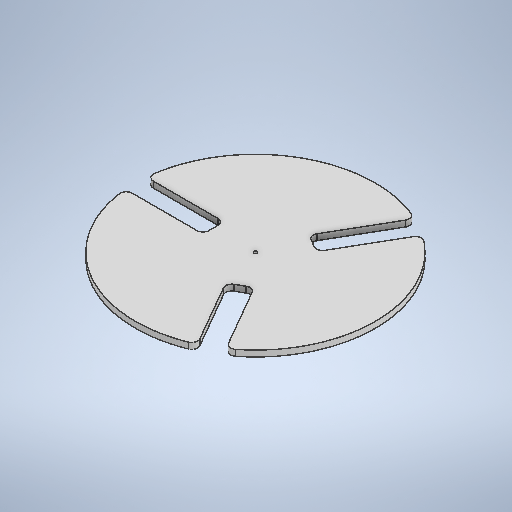
# Autodesk Inventor part: RT_FRM_V2_MC_004_TopDynamicsPlate
Saved by Autodesk Inventor 2025.3 (Build 293356000, 356)
## iProperties
Created: 2026-04-28
Part Number: RT_FRM_V2_MC_004_TopDynamicsPlate
Material: Generic
Document SubType Name: Modeling
Designer: louis
Density: 1 g/cm^3
Appearance: Default
Mass: 556.266 g
Surface Area: 1307.88 cm^2
Volume: 556.266 cm^3
Author: louis
Autodesk Inventor part; units mm, degrees
ref_plane "YZ Plane" through (0, 0, 0) normal (1, 0, 0) x (0, 1, 0)
ref_plane "XZ Plane" through (0, 0, 0) normal (0, 1, 0) x (-1, 0, 0)
ref_plane "XY Plane" through (0, 0, 0) normal (0, 0, 1) x (1, 0, 0)
sketch "Sketch1" plane through (0, 0, 0) normal (0, 1, 0) x (-1, 0, 0)
  line L0 (30, -2.5) -> (140, -2.5)
  line L1 (185, 0) -> (25, 0)
  line L2 (0, 0) -> (25, 0)
  circle A0 centre (0, 0) radius 200
  line L3 (50, 0) -> (103.8137, 0) construction
  line L4 (105, 16.5) -> (105, 0) construction
  line L5 (105, 66.5) -> (105, 16.5) construction
  line L6 (199.2329, -17.5) -> (70, -17.5)
  line L7 (70, -17.5) -> (70, 17.5)
  line L8 (70, 17.5) -> (199.2329, 17.5)
  line L9 (199.2329, 17.5) -> (199.2329, -17.5)
  line L10 (0, 0) -> (0, 200)
  line L11 (-64.9519, 112.5) -> (0, 0)
  circle A1 centre (0, 0) radius 310 construction
  line L12 (-310, -390) -> (-310, -310) construction
  line L13 (-310, -310) -> (-390, -310) construction
  line L14 (-390, -310) -> (-390, -390) construction
  line L15 (-390, -390) -> (-310, -390) construction
  line L16 (-310, -390) -> (-390, -310) construction
  line L17 (-310, -310) -> (-390, -390) construction
  line L18 (-310, 310) -> (-310, 390) construction
  line L19 (-310, 390) -> (-390, 390) construction
  line L20 (-390, 390) -> (-390, 310) construction
  line L21 (-390, 310) -> (-310, 310) construction
  line L22 (-310, 310) -> (-390, 390) construction
  line L23 (-310, 390) -> (-390, 310) construction
  line L24 (390, 310) -> (390, 390) construction
  line L25 (390, 390) -> (310, 390) construction
  line L26 (310, 390) -> (310, 310) construction
  line L27 (310, 310) -> (390, 310) construction
  line L28 (390, 310) -> (310, 390) construction
  line L29 (390, 390) -> (310, 310) construction
  line L30 (390, -390) -> (390, -310) construction
  line L31 (390, -310) -> (310, -310) construction
  line L32 (310, -310) -> (310, -390) construction
  line L33 (310, -390) -> (390, -390) construction
  line L34 (390, -390) -> (310, -310) construction
  line L35 (390, -310) -> (310, -390) construction
  line L36 (310, -310) -> (310, 310) construction
  line L37 (310, 310) -> (-310, 310) construction
  line L38 (-310, 310) -> (-310, -310) construction
  line L39 (-310, -310) -> (310, -310) construction
  line L40 (-64.9519, 112.5) -> (-100, 173.2051)
  line L41 (160, 17.5) -> (199.2329, 17.5)
  line L42 (-114.7719, 163.7908) -> (-84.461, 181.2908)
  line L43 (-84.461, -181.2908) -> (-114.7719, -163.7908)
  point P0 (188.2651, -67.5)
  point P1 (70, 0)
  point P2 (-84.461, 181.2908)
  point P3 (-99.6165, 172.5408)
  point P4 (199.2329, 0)
  point P5 (-114.7719, 163.7908)
  point P6 (-84.461, -181.2908)
  point P7 (-114.7719, -163.7908)
  dimension "d0" = 110
  dimension "d2" = 2.5
  dimension "d4" = 105
  dimension "d9" = 400
  dimension "d26" = 35
  dimension "d27" = 35
  dimension "d40" = 50
  dimension "d46" = 120
  dimension "d74" = 80
  dimension "d75" = 80
  dimension "d78" = 80
  dimension "d79" = 80
  dimension "d80" = 80
  dimension "d81" = 80
  dimension "d82" = 80
  dimension "d83" = 80
  dimension "d86" = 620
  dimension "d97" = 360
  constraints: 88 end point, 10 parallel, 10 perpendicular, 6 vertical, 5 point on circle, 3 coincident, 3 horizontal, 3 point on line, 3 tangent, 2 centre point, 2 collinear, 1 midpoint, 10 other
  measures "d0" distance of L0.end L0.start
  measures "d2" distance between parallel lines of L0 L1
  measures "d4" distance of L2.start L4.end
  measures "d9" diameter of A0
  measures "d26" distance between parallel lines of L8 L6
  measures "d27" distance between parallel lines of L4 L7
  measures "d40" distance from line of L6 point (188.265, -67.5)
  measures "d46" angle of L11 L2
  measures "d74" distance of L13.end L14.end
  measures "d75" distance of L14.end L12.start
  measures "d78" distance of L19.end L20.end
  measures "d79" distance of L20.end L18.start
  measures "d80" distance of L25.end L26.end
  measures "d81" distance of L26.end L24.start
  measures "d82" distance of L31.end L32.end
  measures "d83" distance of L32.end L30.start
  measures "d86" distance of L26.end L18.start
extrude "Extrusion1" add sketch "Sketch1" against normal blind 10 contours L1 L2 L10 A0 L8 L7 | L11 L40 L42 A0 L10 | A0 L43
pattern_circular "Circular Pattern2" count 3 over 360 about axis through (0, 0, 0) along (0, -1, 0) of "Extrusion1"
extrude "Extrusion2" cut sketch "Sketch1" against normal blind 10 contours L7 L8 L9 L6 | L9 A0
pattern_circular "Circular Pattern1" count 3 over 360 about axis through (0, -10, 0) along (0, 1, 0) of "Extrusion2"
fillet "Fillet1" radius 10 6 edges at (19.8446, -5, 69.3718) (50.1554, -5, -51.8718) (-70, -5, -17.5) (-70, -5, 17.5) (50.1554, -5, 51.8718) (19.8446, -5, -69.3718)
sketch "Sketch2" plane through (0, -10, 0) normal (0, 1, 0) x (1, 0, 0)
  line L0 (20, 310) -> (-20, 310) construction
  line L1 (-20, 310) -> (-20, -310) construction
  line L2 (-20, -310) -> (20, -310) construction
  line L3 (20, -310) -> (20, 310) construction
  line L4 (20, 310) -> (-20, -310) construction
  line L5 (-20, 310) -> (20, -310) construction
  line L6 (60, 20) -> (20, 20) construction
  line L7 (20, 20) -> (20, -20) construction
  line L8 (20, -20) -> (60, -20) construction
  line L9 (60, -20) -> (60, 20) construction
  line L10 (60, 20) -> (20, -20) construction
  line L11 (20, 20) -> (60, -20) construction
  line L12 (-60, 123.6771) -> (-20, 123.6771) construction
  line L13 (-20, 123.6771) -> (-20, 83.6771) construction
  line L14 (-20, 83.6771) -> (-60, 83.6771) construction
  line L15 (-60, 83.6771) -> (-60, 123.6771) construction
  line L16 (-60, 123.6771) -> (-20, 83.6771) construction
  line L17 (-20, 123.6771) -> (-60, 83.6771) construction
  line L18 (-60, -66.8914) -> (-20, -66.8914) construction
  line L19 (-20, -66.8914) -> (-20, -106.8914) construction
  line L20 (-20, -106.8914) -> (-60, -106.8914) construction
  line L21 (-60, -106.8914) -> (-60, -66.8914) construction
  line L22 (-60, -66.8914) -> (-20, -106.8914) construction
  line L23 (-20, -66.8914) -> (-60, -106.8914) construction
  point P0 (0, 0)
  point P1 (40, 0)
  point P2 (-40, 103.6771)
  point P3 (-40, -86.8914)
  dimension "d87" = 40
  dimension "d88" = 620
  dimension "d89" = 40
  dimension "d90" = 40
  dimension "d91" = 40
  dimension "d92" = 40
  dimension "d93" = 40
  dimension "d94" = 40
  constraints: 48 end point, 8 midpoint, 8 parallel, 4 horizontal, 4 perpendicular, 3 collinear
  measures "d87" distance of L2.end L1.end
  measures "d88" distance of L1.end L0.end
  measures "d89" distance of L8.end L7.end
  measures "d90" distance of L7.end L6.end
  measures "d91" distance of L13.end L14.end
  measures "d92" distance of L19.end L20.end
  measures "d93" distance of L18.end L19.end
  measures "d94" distance of L14.end L12.start
hole "Hole2" [suppressed]
sketch "Sketch3" plane through (0, -10, 0) normal (0, -1, 0) x (1, 0, 0)
  point P0 (0, 0)
  point P1 (0, 0)
  constraints: 1 coincident
hole "Hole3" at (0, -10, 0) direction (0, 1, 0) diameter 5.5 end through all start extended yes counterbore diameter 10 counterbore depth 5 clearance for "Socket Head Cap Screw" size "M5" standard "Ansi Metric M Profile"
fillet "Fillet2" radius 10 6 edges at (84.461, -5, -181.2908) (114.7719, -5, -163.7908) (114.7719, -5, 163.7908) (84.461, -5, 181.2908) (-199.2329, -5, -17.5) (-199.2329, -5, 17.5)
body "Solid1"
